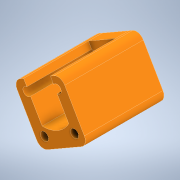
# Autodesk Inventor part: n20 motor 3dp support
Saved by Autodesk Inventor 2021 (Build 250183000, 183)
## iProperties
Created: 2021-03-22
Part Number: n20 motor 3dp support
Material: Generic
Document SubType Name: Modeling
Designer: ASUS
Density: 1 g/cm^3
Appearance: Orange
Author: ASUS
Autodesk Inventor part; units mm, degrees
ref_plane "YZ Plane" through (0, 0, 0) normal (1, 0, 0) x (0, 1, 0)
ref_plane "XZ Plane" through (0, 0, 0) normal (0, 1, 0) x (-1, 0, 0)
ref_plane "XY Plane" through (0, 0, 0) normal (0, 0, 1) x (1, 0, 0)
ref_plane "Work Plane1" through (4.3625, 2.5299, 40) normal (0, 0, -1) x (-1, 0, 0)
sketch "Sketch1" plane through (4.3625, 2.5299, 40) normal (0, 0, -1) x (-1, 0, 0)
  arc A0 (17.1224, 1.6801) -> (15.652, 7.1425) centre (13.656, 3.6761) ccw projected
  line L0 (15.652, 7.1425) -> (-1.6801, 17.1224) projected
  arc A1 (-1.6801, 17.1224) -> (-7.1425, 15.652) centre (-3.6761, 13.656) ccw projected
  line L1 (-7.1425, 15.652) -> (-17.1224, -1.6801) projected
  arc A2 (-17.1224, -1.6801) -> (-15.652, -7.1425) centre (-13.656, -3.6761) ccw projected
  line L2 (-15.652, -7.1425) -> (1.6801, -17.1224) projected
  arc A3 (1.6801, -17.1224) -> (7.1425, -15.652) centre (3.6761, -13.656) ccw projected
  line L3 (17.1224, 1.6801) -> (7.1425, -15.652) projected
  circle A4 centre (0, 0) radius 5 projected
  circle A5 centre (-3.2492, 12.0703) radius 2 projected
  circle A6 centre (3.2492, -12.0703) radius 2 projected
  circle A7 centre (-12.0703, -3.2492) radius 2 projected
  circle A8 centre (12.0703, 3.2492) radius 2 projected
  circle A9 centre (-3.2492, 12.0703) radius 2 projected
  circle A10 centre (-12.0703, -3.2492) radius 2 projected
  circle A11 centre (3.2492, -12.0703) radius 2 projected
  circle A12 centre (12.0703, 3.2492) radius 2 projected
  circle A13 centre (0.0668, -0.0564) radius 2 projected
  circle A14 centre (-3.1634, -1.6582) radius 0.5 projected
  circle A15 centre (3.297, 1.5455) radius 0.5 projected
  arc A16 (-1.6801, 17.1224) -> (-7.1425, 15.652) centre (-3.6761, 13.656) ccw projected
  line L4 (15.652, 7.1425) -> (-1.6801, 17.1224) projected
  arc A17 (17.1224, 1.6801) -> (15.652, 7.1425) centre (13.656, 3.6761) ccw projected
  line L5 (7.1425, -15.652) -> (17.1224, 1.6801) projected
  arc A18 (1.6801, -17.1224) -> (7.1425, -15.652) centre (3.6761, -13.656) ccw projected
  line L6 (1.6801, -17.1224) -> (-15.652, -7.1425) projected
  arc A19 (-17.1224, -1.6801) -> (-15.652, -7.1425) centre (-13.656, -3.6761) ccw projected
  line L7 (-17.1224, -1.6801) -> (-7.1425, 15.652) projected
  circle A20 centre (-3.2492, 12.0703) radius 2 projected
  circle A21 centre (-12.0703, -3.2492) radius 2 projected
  circle A22 centre (3.2492, -12.0703) radius 2 projected
  circle A23 centre (12.0703, 3.2492) radius 2 projected
  circle A24 centre (0.0668, -0.0564) radius 2 projected
  circle A25 centre (-3.1634, -1.6582) radius 0.5 projected
  circle A26 centre (3.297, 1.5455) radius 0.5 projected
  arc A27 (-1.6801, 17.1224) -> (-7.1425, 15.652) centre (-3.6761, 13.656) ccw projected
  line L8 (15.652, 7.1425) -> (-1.6801, 17.1224) projected
  arc A28 (17.1224, 1.6801) -> (15.652, 7.1425) centre (13.656, 3.6761) ccw projected
  line L9 (7.1425, -15.652) -> (17.1224, 1.6801) projected
  arc A29 (1.6801, -17.1224) -> (7.1425, -15.652) centre (3.6761, -13.656) ccw projected
  line L10 (1.6801, -17.1224) -> (-15.652, -7.1425) projected
  arc A30 (-17.1224, -1.6801) -> (-15.652, -7.1425) centre (-13.656, -3.6761) ccw projected
  line L11 (-17.1224, -1.6801) -> (-7.1425, 15.652) projected
  circle A31 centre (-3.2492, 12.0703) radius 2 projected
  circle A32 centre (-12.0703, -3.2492) radius 2 projected
  circle A33 centre (3.2492, -12.0703) radius 2 projected
  circle A34 centre (12.0703, 3.2492) radius 2 projected
  circle A35 centre (0.0668, -0.0564) radius 2 projected
  circle A36 centre (-3.1634, -1.6582) radius 0.5 projected
  circle A37 centre (3.297, 1.5455) radius 0.5 projected
  arc A38 (-1.6801, 17.1224) -> (-7.1425, 15.652) centre (-3.6761, 13.656) ccw projected
  line L12 (15.652, 7.1425) -> (-1.6801, 17.1224) projected
  arc A39 (17.1224, 1.6801) -> (15.652, 7.1425) centre (13.656, 3.6761) ccw projected
  line L13 (7.1425, -15.652) -> (17.1224, 1.6801) projected
  arc A40 (1.6801, -17.1224) -> (7.1425, -15.652) centre (3.6761, -13.656) ccw projected
  line L14 (1.6801, -17.1224) -> (-15.652, -7.1425) projected
  arc A41 (-17.1224, -1.6801) -> (-15.652, -7.1425) centre (-13.656, -3.6761) ccw projected
  line L15 (-17.1224, -1.6801) -> (-7.1425, 15.652) projected
  circle A42 centre (-3.2492, 12.0703) radius 2 projected
  circle A43 centre (-12.0703, -3.2492) radius 2 projected
  circle A44 centre (3.2492, -12.0703) radius 2 projected
  circle A45 centre (12.0703, 3.2492) radius 2 projected
  circle A46 centre (0.0668, -0.0564) radius 2 projected
  circle A47 centre (-3.1634, -1.6582) radius 0.5 projected
  circle A48 centre (3.297, 1.5455) radius 0.5 projected
  arc A49 (-1.6801, 17.1224) -> (-7.1425, 15.652) centre (-3.6761, 13.656) ccw projected
  line L16 (15.652, 7.1425) -> (-1.6801, 17.1224) projected
  arc A50 (17.1224, 1.6801) -> (15.652, 7.1425) centre (13.656, 3.6761) ccw projected
  line L17 (7.1425, -15.652) -> (17.1224, 1.6801) projected
  arc A51 (1.6801, -17.1224) -> (7.1425, -15.652) centre (3.6761, -13.656) ccw projected
  line L18 (1.6801, -17.1224) -> (-15.652, -7.1425) projected
  arc A52 (-17.1224, -1.6801) -> (-15.652, -7.1425) centre (-13.656, -3.6761) ccw projected
  line L19 (-17.1224, -1.6801) -> (-7.1425, 15.652) projected
  line L20 (1.3233, 4.8217) -> (-9.7179, 11.1793)
  line L21 (4.3625, -2.5299) -> (12.1325, -6.9859) construction
  line L22 (-3.5176, -3.6192) -> (-14.5807, 2.7001)
  dimension "d1" = 4
  constraints: 6 end point, 2 symmetric about line, 1 midpoint, 1 parallel, 1 point on line, 2 other
  measures "d1" distance from line of L20 A9.centre
ref_plane "Work Plane2" through (-14.2412, -15.9727, 0) normal (0, 0, 1) x (1, 0, 0)
extrude "Extrusion1" add sketch "Sketch1" along normal up to surface (40 mm away) contours L3 A3 L2 A2 L1 A1 L0 A0
sketch "Sketch2" plane through (4.3625, 2.5299, 40) normal (0, 0, 1) x (1, 0, 0)
  line L0 (-15.652, 7.1425) -> (1.6801, 17.1224) projected
  circle A0 centre (3.2492, 12.0703) radius 2 projected
  circle A1 centre (-12.0703, 3.2492) radius 2 projected
  line L1 (9.2077, -0.2818) -> (-0.1928, 16.044)
  line L2 (-4.3786, -8.1049) -> (-13.7791, 8.2209)
  line L3 (-4.3786, -8.1049) -> (9.2077, -0.2818)
  circle A2 centre (12.0703, -3.2492) radius 2 projected
  circle A3 centre (-3.2492, -12.0703) radius 2 projected
  point P0 (-4.3625, -2.5299)
  point P1 (3.2469, 10.0703)
  point P2 (1.5183, 13.0723)
  point P3 (-12.068, 5.2492)
  point P4 (-10.3394, 2.2472)
  dimension "d6" = 1
  dimension "d7" = 1
  dimension "d8" = 4
  constraints: 6 end point, 2 parallel, 2 point on line, 1 perpendicular
  measures "d6" distance from line of L1 A0.centre
  measures "d7" distance from line of A1.centre L2
  measures "d8" distance from line of A2.centre L3
extrude "Extrusion2" cut sketch "Sketch2" against normal up to surface (40 mm away) contours L0 L1 A0 L3 L2 A1
sketch "Sketch3" plane through (4.3625, 2.5299, 40) normal (0, 0, 1) x (1, 0, 0)
  arc A0 (1.3233, -4.8217) -> (3.5058, -3.565) centre (0, 0) ccw projected
  line L0 (1.3233, -4.8217) -> (3.5058, -3.565)
  point P0 (-4.3625, -2.5299)
  constraints: 2 end point
extrude "Extrusion3" add sketch "Sketch3" against normal up to surface (40 mm away)
sketch "Sketch4" plane through (4.3625, 2.5299, 40) normal (0, 0, 1) x (1, 0, 0)
  line L0 (-4.3786, -8.1049) -> (9.2077, -0.2818) projected
  arc A0 (-4.3786, -8.1049) -> (9.2077, -0.2818) centre (-3.967, 6.8895) ccw
  point P0 (-4.3625, -2.5299)
  dimension "d14" = 15
  constraints: 2 point on circle, 1 centre point
  measures "d14" radius of A0
extrude "Extrusion4" cut sketch "Sketch4" against normal up to surface (40 mm away)
sketch "Sketch5" plane through (21.485, 0.8498, 0) normal (0, 0, -1) x (-0.8666046, -0.4989954, 0)
  line L0 (6.1612, 17.1068) -> (6.1612, 17.1068) projected
  arc A0 (6.1612, 20.5709) -> (6.1612, 17.1068) centre (5.1612, 18.8388) ccw projected
  arc A1 (6.1612, 17.1068) -> (6.1612, 20.5709) centre (5.1612, 18.8388) ccw
  line L1 (21.8388, 24) -> (21.8388, 20.5709) projected
  line L2 (21.8388, 17.1068) -> (21.8388, 17.1068) projected
  arc A2 (21.8388, 20.5709) -> (21.8388, 17.1068) centre (22.8388, 18.8388) ccw
  arc A3 (21.8388, 17.1068) -> (21.8388, 20.5709) centre (22.8388, 18.8388) ccw projected
  line L3 (21.8388, 17.1068) -> (21.8388, 5.1612) projected
  line L4 (21.8388, 14) -> (6.1612, 14)
  line L5 (24, 24) -> (21.8388, 24) projected
  line L6 (6.1612, 24) -> (4, 24) projected
  line L7 (21.8388, 24) -> (6.1612, 24)
  line L8 (6.1612, 5.1612) -> (6.1612, 17.1068) projected
  line L9 (6.1612, 20.5709) -> (6.1612, 24) projected
  point P0 (19.043, 9.9845)
  dimension "d17" = 10
  constraints: 5 point on circle, 4 end point, 2 centre point, 2 coincident, 1 collinear, 1 horizontal, 1 point on line
  measures "d17" distance from line of L1.start L4
extrude "Extrusion5" add sketch "Sketch5" against normal blind 7 contours L9 L7 L1 A2 L3 L4 L8 A1
sketch "Sketch6" plane through (21.485, 0.8498, 0) normal (0, 0, -1) x (-0.8666046, -0.4989954, 0)
  line L0 (21.8388, 14) -> (21.8388, 5.1612) projected
  arc A0 (6.1612, 5.1612) -> (21.8388, 5.1612) centre (14, 17.9499) ccw projected
  line L1 (6.1612, 5.1612) -> (6.1612, 14) projected
  line L2 (6.1612, 14) -> (21.8388, 14) projected
  arc A1 (21.8388, 20.5709) -> (21.8388, 17.1068) centre (22.8388, 18.8388) ccw construction
  arc A2 (21.8388, 17.1068) -> (21.8388, 20.5709) centre (22.8388, 18.8388) ccw projected
  line L3 (21.8388, 24) -> (6.1612, 24) projected
  line L4 (6.1612, 24) -> (4, 24) projected
  arc A3 (4, 24) -> (0, 20) centre (4, 20) ccw projected
  line L5 (0, 20) -> (0, 0) projected
  arc A4 (0, 0) -> (4, -4) centre (4, 0) ccw projected
  line L6 (4, -4) -> (24, -4) projected
  arc A5 (24, -4) -> (28, 0) centre (24, 0) ccw projected
  line L7 (28, 0) -> (28, 20) projected
  arc A6 (28, 20) -> (24, 24) centre (24, 20) ccw projected
  line L8 (24, 24) -> (21.8388, 24) projected
  arc A7 (6.1612, 17.1068) -> (6.1612, 20.5709) centre (5.1612, 18.8388) ccw projected
  arc A8 (6.1612, 20.5709) -> (6.1612, 17.1068) centre (5.1612, 18.8388) ccw construction
  circle A9 centre (22.8388, 1.1612) radius 2 projected
  circle A10 centre (5.1612, 1.1612) radius 2 projected
  circle A11 centre (22.8388, 1.1612) radius 2 projected
  circle A12 centre (22.8388, 1.1612) radius 2.1
  circle A13 centre (5.1612, 1.1612) radius 2.1
  arc A14 (6.1612, 17.1068) -> (6.1612, 20.5709) centre (5.1612, 18.8388) ccw projected
  circle A15 centre (5.1612, 18.8388) radius 2.1
  arc A16 (21.8388, 17.1068) -> (21.8388, 20.5709) centre (22.8388, 18.8388) ccw projected
  circle A17 centre (22.8388, 18.8388) radius 2.1
  point P0 (19.043, 9.9845)
  dimension "d20" = 4.2
  constraints: 4 centre point, 4 coincident, 3 equal radius
  measures "d20" diameter of A15
extrude "Extrusion6" cut sketch "Sketch6" against normal up to surface (40 mm away) contours A10 | A12 | A13 | A15 | A17
equation "\"d7\" = d6"
body "Solid1"
